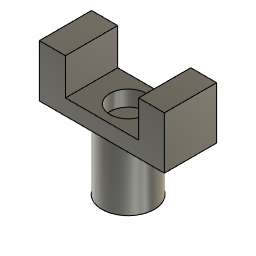
RadioButton (Autodesk Fusion 360 design; units mm, degrees)
Autodesk Fusion 360 part; units mm, degrees
sketch "Sketch1" plane through (0, 0, 0) normal (0, 0, 1) x (1, 0, 0)
  circle A0 centre (0, 0) radius 2.5
  dimension "d1" = 5
  constraint coincident A0.centre origin
  measures "d1" diameter of A0
extrude "Extrude1" add sketch "Sketch1" along normal blind 6
sketch "Sketch2" plane through (0, 0, 6) normal (0, 0, 1) x (-1, 0, 0)
  circle A0 centre (0, 0) radius 2.5
  circle A1 centre (0, 0) radius 1.75
  line L0 (0.0241, -1.7498) -> (0.0241, -2.4999)
  line L1 (1.75, 0) -> (2.5, 0)
  line L2 (2.5, 0) -> (4.5, 0)
  line L3 (0.0241, -2.4999) -> (4.5, -2.4999)
  line L4 (4.5, -2.4999) -> (4.5, 0)
  line L5 (4.5, 0) -> (0.0241, 0)
  line L6 (0.0241, 0) -> (0.0241, -2.4999)
  line L7 (0, 0) -> (4.5, 0)
  line L8 (4.5, 0) -> (4.5, 2.5)
  line L9 (4.5, 2.5) -> (0, 2.5)
  line L10 (0, 2.5) -> (0, 0)
  line L11 (0.0241, -2.4999) -> (-4.4759, -2.4999)
  line L12 (-4.4759, -2.4999) -> (-4.4759, 0)
  line L13 (-4.4759, 0) -> (0.0241, 0)
  line L14 (0.0241, 0) -> (0.0241, -2.4999)
  line L15 (-4.4759, -2.4999) -> (4.5, -2.4999)
  line L16 (4.5, -2.4999) -> (4.5, 2.5)
  line L17 (4.5, 2.5) -> (-4.4759, 2.5)
  line L18 (-4.4759, 2.5) -> (-4.4759, -2.4999)
  dimension "d4" = 3.5
  dimension "d5" = 2
  dimension "d6" = 4.5
  constraint concentric A0 A1
  constraint coincident A1 L0.start
  constraint coincident A0 L0.end
  constraint vertical L0
  constraint coincident A1 L1.start
  constraint coincident A0 L1.end
  constraint perpendicular L0 L1
  constraint parallel L1 L2
  constraint horizontal L3
  constraint vertical L4
  constraint horizontal L5
  constraint vertical L6
  constraint horizontal L7
  constraint vertical L8
  constraint horizontal L9
  constraint vertical L10
  constraint coincident A0.centre A1.centre
  constraint horizontal L11
  constraint vertical L12
  constraint horizontal L13
  constraint vertical L14
  constraint horizontal L15
  constraint vertical L16
  constraint horizontal L17
  constraint vertical L18
  measures "d4" diameter of A1
  measures "d5" distance of L1.end L2.end
  measures "d6" distance of L0.end L11.end
extrude "Extrude2" add sketch "Sketch2" along normal blind 1.5 contours A0 A1 L1 L5 L7 L10 | A0 L2 L3 L4 L5 L7 L15 L16 | A0 A1 L0 L1 L5 L6 L7 L14 | A0 L2 L5 L7 L8 L9 L16 L17 | A0 A1 L10 L13 | A0 L11 L12 L13 L15 L18 | A0 L13 L17 L18 | A0 A1 L0 L6 L13 L14
sketch "Sketch3" plane through (0, 0, 7.5) normal (0, 0, 1) x (-1, 0, 0)
  circle A0 centre (0, 0) radius 1.75
  line L0 (-4.4759, 2.5) -> (-4.4759, -2.4999)
  line L1 (-4.4759, -2.4999) -> (4.5, -2.4999)
  line L2 (4.5, -2.4999) -> (4.5, 2.5)
  line L3 (4.5, 2.5) -> (-4.4759, 2.5)
  line L4 (0, 0) -> (3.5, 0)
  line L5 (3.5, 0) -> (3.5, -2.4999)
  line L6 (3.5, -2.4999) -> (0, -2.4999)
  line L7 (0, -2.4999) -> (0, 0)
  line L8 (3.5, -2.4999) -> (-3.5, -2.4999)
  line L9 (-3.5, -2.4999) -> (-3.5, 2.5)
  line L10 (-3.5, 2.5) -> (3.5, 2.5)
  line L11 (3.5, 2.5) -> (3.5, -2.4999)
  dimension "d9" = 3.5
  dimension "d10" = 7
  constraint horizontal L4
  constraint vertical L5
  constraint horizontal L6
  constraint vertical L7
  constraint coincident A0.centre L4.start
  constraint horizontal L8
  constraint vertical L9
  constraint horizontal L10
  constraint vertical L11
  measures "d9" distance of A0.centre L4.end
  measures "d10" distance of L5.end L8.end
extrude "Extrude3" add sketch "Sketch3" along normal blind 3.5 contours L1 L2 L3 L5 L11 | L0 L1 L3 L9
extrude "Extrude4" add 2 faces at (-4.5, -0.8333, 6.5) (-4.5, 0, 9.8333) along direction (-1, 0, 0) blind 1.5
extrude "Extrude5" add 1 faces at (4.4759, 0.8333, 7.6667) along direction (1, 0, 0) blind 1.5
